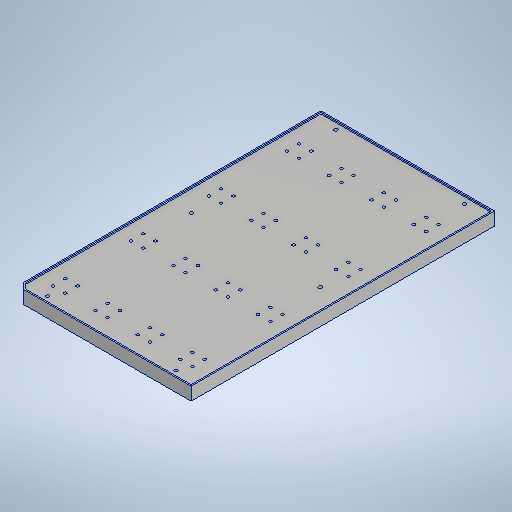
# Autodesk Inventor part: Assembly Plate
Saved by Autodesk Inventor 2025 (Build 290162000, 162)
## iProperties
Created: 2021-01-11
Part Number: Assembly Plate
Material: Aluminum 6061
Document SubType Name: Modeling
Designer: caleb
Density: 2.7 g/cm^3
Appearance: Aluminum - Flat
Author: caleb
Autodesk Inventor part; units mm, degrees
ref_plane "YZ Plane" through (0, 0, 0) normal (1, 0, 0) x (0, 1, 0)
ref_plane "XZ Plane" through (0, 0, 0) normal (0, 1, 0) x (-1, 0, 0)
ref_plane "XY Plane" through (0, 0, 0) normal (0, 0, 1) x (1, 0, 0)
sketch "Sketch1" plane through (0, 0, 0) normal (0, 1, 0) x (-1, 0, 0)
  line L0 (-63.5, 111) -> (63.5, 111)
  line L1 (63.5, 111) -> (63.5, -111)
  line L2 (63.5, -111) -> (-63.5, -111)
  line L3 (-63.5, -111) -> (-63.5, 111)
  line L4 (-63.5, 111) -> (63.5, -111) construction
  line L5 (63.5, 111) -> (-63.5, -111) construction
  point P0 (0, 0)
  dimension "d0" = 127
  dimension "d1" = 222
  constraints: 12 end point, 2 midpoint, 2 parallel, 1 horizontal, 1 perpendicular
  measures "d0" distance of L1.end L2.end
  measures "d1" distance of L0.end L1.end
extrude "Extrusion1" add sketch "Sketch1" along normal blind 9.525
chamfer "Chamfer1" distance 4.5 angle 45 1 edges at (-63.5, 4.7625, 111)
sketch "Sketch10" plane through (0, 9.525, 0) normal (0, 1, 0) x (1, 0, 0)
  circle A0 centre (-51.5, -97) radius 1
  circle A1 centre (-51.5, -88) radius 1
  circle A2 centre (-42.5, -97) radius 1
  circle A3 centre (-42.5, -88) radius 1
  line L0 (-63.5, 111) -> (-63.5, -106.5) projected
  line L1 (-59, -111) -> (63.5, -111) projected
  circle A4 centre (-51.5, -40) radius 1
  circle A5 centre (-51.5, -31) radius 1
  circle A6 centre (-42.5, -40) radius 1
  circle A7 centre (-42.5, -31) radius 1
  circle A8 centre (-51.5, 17) radius 1
  circle A9 centre (-51.5, 26) radius 1
  circle A10 centre (-42.5, 17) radius 1
  circle A11 centre (-42.5, 26) radius 1
  circle A12 centre (-51.5, 74) radius 1
  circle A13 centre (-51.5, 83) radius 1
  circle A14 centre (-42.5, 74) radius 1
  circle A15 centre (-42.5, 83) radius 1
  circle A16 centre (-20.5, -97) radius 1
  circle A17 centre (-20.5, -88) radius 1
  circle A18 centre (-11.5, -97) radius 1
  circle A19 centre (-11.5, -88) radius 1
  circle A20 centre (-20.5, -40) radius 1
  circle A21 centre (-20.5, -31) radius 1
  circle A22 centre (-11.5, -40) radius 1
  circle A23 centre (-11.5, -31) radius 1
  circle A24 centre (-20.5, 17) radius 1
  circle A25 centre (-20.5, 26) radius 1
  circle A26 centre (-11.5, 17) radius 1
  circle A27 centre (-11.5, 26) radius 1
  circle A28 centre (-20.5, 74) radius 1
  circle A29 centre (-20.5, 83) radius 1
  circle A30 centre (-11.5, 74) radius 1
  circle A31 centre (-11.5, 83) radius 1
  line L2 (63.5, 111) -> (-63.5, 111) projected
  circle A32 centre (10.5, -97) radius 1
  circle A33 centre (10.5, -88) radius 1
  circle A34 centre (19.5, -97) radius 1
  circle A35 centre (19.5, -88) radius 1
  circle A36 centre (10.5, -40) radius 1
  circle A37 centre (10.5, -31) radius 1
  circle A38 centre (19.5, -40) radius 1
  circle A39 centre (19.5, -31) radius 1
  circle A40 centre (10.5, 17) radius 1
  circle A41 centre (10.5, 26) radius 1
  circle A42 centre (19.5, 17) radius 1
  circle A43 centre (19.5, 26) radius 1
  circle A44 centre (10.5, 74) radius 1
  circle A45 centre (10.5, 83) radius 1
  circle A46 centre (19.5, 74) radius 1
  circle A47 centre (19.5, 83) radius 1
  circle A48 centre (41.5, -97) radius 1
  circle A49 centre (41.5, -88) radius 1
  circle A50 centre (50.5, -97) radius 1
  circle A51 centre (50.5, -88) radius 1
  circle A52 centre (41.5, -40) radius 1
  circle A53 centre (41.5, -31) radius 1
  circle A54 centre (50.5, -40) radius 1
  circle A55 centre (50.5, -31) radius 1
  circle A56 centre (41.5, 17) radius 1
  circle A57 centre (41.5, 26) radius 1
  circle A58 centre (50.5, 17) radius 1
  circle A59 centre (50.5, 26) radius 1
  circle A60 centre (41.5, 74) radius 1
  circle A61 centre (41.5, 83) radius 1
  circle A62 centre (50.5, 74) radius 1
  circle A63 centre (50.5, 83) radius 1
  point P0 (0, 0)
  dimension "d129" = 2
  dimension "d130" = 9
  dimension "d131" = 9
  dimension "d134" = 12
  dimension "d135" = 14
  dimension "d140" = 57
  dimension "d143" = 31
  dimension "d176" = 28
  constraints: 64 centre point, 3 equal radius, 2 horizontal alignment, 2 vertical alignment, 1 horizontal, 1 vertical, 120 other
  measures "d129" diameter of A0
  measures "d130" distance of A0.centre A1.centre
  measures "d131" distance of A2.centre A0.centre
  measures "d134" distance from line of L0 A0.centre
  measures "d135" distance from line of L1 A0.centre
  measures "d140" distance of A0.centre A4.centre
  measures "d143" distance of A0.centre A16.centre
  measures "d176" distance from line of L2 A13.centre
extrude "Extrusion8" cut sketch "Sketch10" against normal through all
sketch "Sketch12" plane through (0, 9.525, 0) normal (0, 1, 0) x (1, 0, 0)
  line L0 (62.5, 110) -> (-62.5, 110)
  line L1 (-62.5, 110) -> (-62.5, -106.0858)
  line L2 (-58.5858, -110) -> (62.5, -110)
  line L3 (62.5, -110) -> (62.5, 110)
  line L4 (-63.5, 111) -> (-63.5, -106.5) projected
  line L5 (63.5, 111) -> (-63.5, 111) projected
  line L6 (63.5, -111) -> (63.5, 111) projected
  line L7 (-59, -111) -> (63.5, -111) projected
  line L8 (-62.5, -106.0858) -> (-58.5858, -110)
  line L9 (-59, -111) -> (-63.5, -106.5) projected
  point P0 (0, 0)
  point P1 (-62.5, -110)
  dimension "d166" = 1
  dimension "d167" = 1
  dimension "d168" = 1
  dimension "d169" = 1
  dimension "d177" = 1
  constraints: 10 end point, 2 parallel, 2 point on line, 1 horizontal, 1 perpendicular
  measures "d166" distance between parallel lines of L4 L1
  measures "d167" distance between parallel lines of L5 L0
  measures "d168" distance between parallel lines of L6 L3
  measures "d169" distance between parallel lines of L7 L2
  measures "d177" distance between parallel lines of L9 L8
extrude "Extrusion10" cut sketch "Sketch12" against normal blind 1 contours L3 L2 L8 L1 L0
fillet "Fillet3" radius 1 5 edges at (62.5, 9.025, -110) (-58.5858, 9.025, 110) (-62.5, 9.025, 106.0858) (62.5, 9.025, 110) (-62.5, 9.025, -110)
sketch "Sketch13" plane through (0, 8.525, 0) normal (0, 1, 0) x (1, 0, 0)
  line L0 (-62.5, -105.6716) -> (-62.5, 109) projected
  line L1 (62.5, 109) -> (62.5, -109) projected
  line L2 (61.5, -110) -> (-58.1716, -110) projected
  line L3 (-61.5, 110) -> (61.5, 110) projected
  point P0 (0, 0)
  point P1 (-47, -105.5)
  point P2 (47, -105.5)
  point P3 (-47, 0)
  point P4 (47, 0)
  point P5 (-47, 105.5)
  point P6 (47, 105.5)
  dimension "d178" = 15.5
  dimension "d179" = 15.5
  dimension "d180" = 4.5
  dimension "d181" = 4.5
  constraints: 4 horizontal alignment, 4 vertical alignment
  measures "d178" distance from line of point (-47, -105.5) L0
  measures "d179" distance from line of L1 point (47, -105.5)
  measures "d180" distance from line of L2 point (47, -105.5)
  measures "d181" distance from line of L3 point (-47, 105.5)
hole "Hole3" at (-47, 8.525, 105.5) at (47, 8.525, 105.5) at (-47, 8.525, 0) at (47, 8.525, 0) at (-47, 8.525, -105.5) at (47, 8.525, -105.5) direction (0, -1, 0) diameter 2.459 depth 8.8 tip angle 118 thread size "M3x0.5" class "6H" standard "ANSI Metric M Profile"
body "Solid1"
